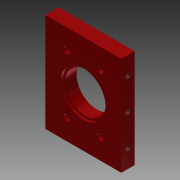
# Autodesk Inventor part: Swerve Wheel + Carriage Outline V1
Saved by Autodesk Inventor 2013 (Build 170138000, 138)
## iProperties
Created: 2013-04-01
Part Number: Swerve Wheel + Carriage Outline V1
Material: Generic
Document SubType Name: Sheet Metal
Designer: mvarma
Density: 1 g/cm^3
Sheet Metal Rule: Default
Author: mvarma
Autodesk Inventor part; units mm, degrees
ref_plane "YZ Plane" through (0, 0, 0) normal (1, 0, 0) x (0, 1, 0)
ref_plane "XZ Plane" through (0, 0, 0) normal (0, 1, 0) x (-1, 0, 0)
sketch "Sketch1" plane through (0, 0, 0) normal (0, 0, 1) x (1, 0, 0)
  circle A0 centre (0, 0) radius 38.1 construction
  circle A1 centre (0, 0) radius 41.275 construction
  line L0 (-7.3323, 0) -> (-3.6662, 6.35) construction
  line L1 (-3.6662, 6.35) -> (3.6662, 6.35) construction
  line L2 (3.6662, 6.35) -> (7.3323, 0) construction
  line L3 (7.3323, 0) -> (3.6662, -6.35) construction
  line L4 (3.6662, -6.35) -> (-3.6662, -6.35) construction
  line L5 (-3.6662, -6.35) -> (-7.3323, 0) construction
  circle A2 centre (0, 0) radius 14.2875 construction
  circle A3 centre (0, 0) radius 15.875 construction
  circle A4 centre (0, 0) radius 8.7313 construction
  circle A5 centre (0, 0) radius 22.225 construction
  line L6 (34.925, 38.1) -> (34.925, 95.25) construction
  line L7 (34.925, 95.25) -> (-34.925, 95.25) construction
  line L8 (-34.925, 95.25) -> (-34.925, 38.1) construction
  line L9 (34.925, 38.1) -> (-34.925, 38.1) construction
  line L10 (34.925, 38.1) -> (21.2491, -6.5137) construction
  line L11 (-34.925, 38.1) -> (-21.2491, -6.5137) construction
  circle A6 centre (-30.353, 38.1) radius 3.9624 construction
  line L12 (53.34, 95.25) -> (-53.34, 95.25) construction
  line L13 (-53.34, 95.25) -> (-53.34, 104.775) construction
  line L14 (-53.34, 104.775) -> (53.34, 104.775) construction
  line L15 (53.34, 104.775) -> (53.34, 95.25) construction
  circle A7 centre (-222.5199, 24.1494) radius 53.34 construction
  line L16 (-190.7699, 59.0744) -> (-254.2699, 59.0744)
  line L17 (-254.2699, 59.0744) -> (-254.2699, -10.7756)
  line L18 (-254.2699, -10.7756) -> (-190.7699, -10.7756)
  line L19 (-190.7699, -10.7756) -> (-190.7699, 59.0744)
  line L20 (-195.5324, 59.0744) -> (-195.5324, -10.7756)
  line L21 (-249.5074, 59.0744) -> (-249.5074, -10.7756)
  line L22 (-209.8199, 68.5994) -> (-235.2199, 68.5994) construction
  line L23 (-235.2199, 68.5994) -> (-235.2199, -20.3006) construction
  line L24 (-235.2199, -20.3006) -> (-209.8199, -20.3006) construction
  line L25 (-209.8199, -20.3006) -> (-209.8199, 68.5994) construction
  line L26 (34.925, 88.9) -> (-34.925, 88.9) construction
  circle A8 centre (30.353, 38.1) radius 3.9624 construction
  circle A9 centre (30.353, 76.2) radius 3.9624 construction
  circle A10 centre (-30.353, 76.2) radius 3.9624 construction
  circle A11 centre (0, 47.625) radius 3.9624 construction
  line L27 (34.925, 92.075) -> (-34.925, 92.075) construction
  circle A12 centre (0, 71.755) radius 14.2875 construction
  circle A13 centre (0, 71.755) radius 15.875 construction
  line L28 (7.3323, 71.755) -> (3.6662, 65.405) construction
  line L29 (3.6662, 65.405) -> (-3.6662, 65.405) construction
  line L30 (-3.6662, 65.405) -> (-7.3323, 71.755) construction
  line L31 (-7.3323, 71.755) -> (-3.6662, 78.105) construction
  line L32 (-3.6662, 78.105) -> (3.6662, 78.105) construction
  line L33 (3.6662, 78.105) -> (7.3323, 71.755) construction
  point P0 (22.225, 92.075)
  point P1 (0, 92.075)
  point P2 (-22.225, 92.075)
  point P3 (0, 47.625)
  dimension "d0" = 76.2
  dimension "d2" = 82.55
  dimension "d3" = 12.7
  dimension "d4" = 28.575
  dimension "d5" = 31.75
  dimension "d6" = 17.4625
  dimension "d7" = 44.45
  dimension "d8" = 69.85
  dimension "d9" = 34.925
  dimension "d10" = 38.1
  dimension "d11" = 57.15
  dimension "d13" = 7.9248
  dimension "d14" = 9.525
  dimension "d15" = 106.68
  dimension "d16" = 53.34
  dimension "d17" = 106.68
  dimension "d18" = 69.85
  dimension "d19" = 34.925
  dimension "d20" = 63.5
  dimension "d21" = 31.75
  dimension "d22" = 4.7625
  dimension "d23" = 4.7625
  dimension "d24" = 25.4
  dimension "d25" = 14.2875
  dimension "d26" = 88.9
  dimension "d27" = 14.2875
  dimension "d28" = 44.45
  dimension "d29" = 4.572
  dimension "d30" = 6.35
  dimension "d31" = 0
  dimension "d32" = 7.9248
  dimension "d33" = 4.572
  dimension "d34" = 7.9248
  dimension "d35" = 7.9248
  dimension "d36" = 4.572
  dimension "d37" = 4.572
  dimension "d38" = 38.1
  dimension "d39" = 38.1
  dimension "d40" = 7.9248
  dimension "d41" = 9.525
  dimension "d42" = 34.925
  dimension "d44" = 3.175
  dimension "d45" = 34.925
  dimension "d46" = 12.7
  dimension "d47" = 12.7
  dimension "d48" = 28.575
  dimension "d50" = 0
  dimension "d52" = 31.75
  dimension "d53" = 12.7
  dimension "d54" = 17.145
  measures "d0" diameter of A0
  measures "d2" diameter of A1
  measures "d3" distance between parallel lines of L4 L1
  measures "d4" diameter of A2
  measures "d5" diameter of A3
  measures "d6" diameter of A4
  measures "d7" diameter of A5
  measures "d8" distance between parallel lines of L8 L6
  measures "d9" distance from line of point (0, 0) L8
  measures "d10" distance from line of L9 point (0, 0)
  measures "d11" distance of L7.end L8.end
  measures "d13" diameter of A6
  measures "d14" distance of L14.end L12.start
  measures "d15" distance of L13.end L14.end
  measures "d16" horizontal distance of L12.start point (0, 0)
  measures "d17" diameter of A7
  measures "d18" distance of L18.end L16.start
  measures "d19" distance from line of A7.centre L18
  measures "d20" distance of L17.end L18.end
  measures "d21" distance from line of L19 A7.centre
  measures "d22" distance between parallel lines of L17 L21
  measures "d23" distance between parallel lines of L19 L20
  measures "d24" distance between parallel lines of L23 L25
  measures "d25" distance between parallel lines of L20 L25
  measures "d26" distance of L22.end L23.end
  measures "d27" distance between parallel lines of L21 L23
  measures "d28" distance from line of A7.centre L24
  measures "d29" distance from line of L8 A6.centre
  measures "d30" distance between parallel lines of L7 L26
  measures "d31" distance between parallel lines of L7 L12
  measures "d32" diameter of A8
  measures "d33" distance from line of L6 A8.centre
  measures "d34" diameter of A9
  measures "d35" diameter of A10
  measures "d36" distance from line of L8 A10.centre
  measures "d37" distance from line of L6 A9.centre
  measures "d38" distance from line of L9 A10.centre
  measures "d39" distance from line of L9 A9.centre
  measures "d40" diameter of A11
  measures "d41" distance from line of L9 A11.centre
  measures "d42" distance from line of L8 A11.centre
  measures "d44" distance between parallel lines of L26 L27
  measures "d45" distance from line of L8 point (0, 92.075)
  measures "d46" distance from line of L8 point (-22.225, 92.075)
  measures "d47" distance from line of L6 point (22.225, 92.075)
  measures "d48" diameter of A12
  measures "d50" horizontal distance of A11.centre A12.centre
  measures "d52" diameter of A13
  measures "d53" distance between parallel lines of L29 L32
  measures "d54" distance from line of L26 A13.centre
extrude "Plate1" add sketch "Sketch1" along normal blind 9.525 contours L20 L18 L21 L16
sketch "Sketch3" plane through (0, 0, 0) normal (0, 0, -1) x (-1, 0, 0)
  line L0 (249.5074, -10.7756) -> (195.5324, -10.7756) projected
  line L1 (249.5074, 59.0744) -> (249.5074, -10.7756) projected
  circle A0 centre (222.5199, 24.1494) radius 23.8125 construction
  line L2 (210.6137, 44.7716) -> (222.5199, 24.1494) construction
  line L3 (222.5199, 24.1494) -> (198.7074, 24.1494) construction
  point P0 (195.5324, 59.0744)
  point P1 (0, 0)
  point P2 (198.7074, 24.1494)
  point P3 (210.6137, 3.5271)
  point P4 (234.4262, 3.5271)
  point P5 (246.3324, 24.1494)
  point P6 (234.4262, 44.7716)
  dimension "d69" = 47.625
  dimension "d71" = 26.9875
  dimension "d72" = 53.975
  dimension "d73" = 34.925
  dimension "d74" = 69.85
  dimension "d75" = 60
  dimension "d78" = 360
  constraints: 4 end point, 2 point on circle, 1 centre point, 1 coincident, 1 perpendicular, 7 other
  measures "d69" diameter of A0
  measures "d71" distance from line of L1 L2.end
  measures "d72" distance of point (195.532, 59.074) L1.start
  measures "d73" distance from line of L0 L2.end
  measures "d74" distance of L1.start L0.start
  measures "d75" angle of L3 L2
hole "Hole2" at (-210.6137, 44.7716, 0) at (-210.6137, 3.5271, 0) at (-234.4262, 3.5271, 0) at (-234.4262, 44.7716, 0) direction (0, 0, 1) diameter 4.318 end through all counterbore diameter 7.9502 counterbore depth 3.175 clearance for "Socket Head Cap Screw" size "#8" standard "Ansi Unified Screw Threads"
sketch "Sketch4" plane through (0, 0, 9.525) normal (0, 0, 1) x (1, 0, 0)
  line L0 (-249.5074, -10.7756) -> (-249.5074, 59.0744) projected
  line L1 (-195.5324, -10.7756) -> (-249.5074, -10.7756) projected
  point P0 (0, 0)
  point P1 (-222.5199, 24.1494)
  dimension "d97" = 53.975
  dimension "d98" = 69.85
  dimension "d99" = 34.925
  dimension "d100" = 26.9875
  measures "d97" distance of L1.start L0.start
  measures "d98" distance of L0.start L0.end
  measures "d99" distance from line of L1 point (-222.52, 24.149)
  measures "d100" distance from line of L0 point (-222.52, 24.149)
hole "Hole4" at (-222.5199, 24.1494, 9.525) direction (0, 0, -1) diameter 28.575 end through all counterbore diameter 31.75 counterbore depth 1.5875
ref_plane "Work Plane1" through (-222.5199, -10.7756, 0) normal (1, 0, 0) x (0, 0, -1)
sketch "Sketch2" plane through (-195.5324, -10.7756, 0) normal (1, 0, 0) x (0, 0, -1)
  line L0 (0, 0) -> (-9.525, 0) projected
  line L1 (0, 69.85) -> (-9.525, 69.85) projected
  line L2 (-4.7625, 69.85) -> (-4.7625, 0) construction
  point P0 (0, 10.7756)
  point P1 (-4.7625, 57.15)
  point P2 (-4.7625, 34.925)
  point P3 (-4.7625, 12.7)
  dimension "d87" = 12.7
  dimension "d88" = 12.7
  dimension "d89" = 34.925
  constraints: 3 midpoint, 2 end point, 2 point on line
  measures "d87" distance from line of L1 point (-4.763, 57.15)
  measures "d88" distance from line of L0 point (-4.763, 12.7)
  measures "d89" distance from line of L0 point (-4.763, 34.925)
hole "Hole1" at (-195.5324, 46.3744, 4.7625) at (-195.5324, 24.1494, 4.7625) at (-195.5324, 1.9244, 4.7625) direction (-1, 0, 0) diameter 3.9624 depth 7.9375 tip angle 118 thread size "10-32 UNF" class "2B" standard "ANSI Unified Screw Threads"
mirror "Mirror1" about plane through (-222.5199, -10.7756, 0) normal (1, 0, 0) of "Hole1"
equation "\"d99\" = 0.5 * d98"
equation "\"d100\" = 0.5 * d97"
equation "\"d9\" = 0.5 * d8"
equation "\"d16\" = 0.5 * d15"
equation "\"d19\" = 0.5 * d18"
equation "\"d21\" = 0.5 * d20"
equation "\"d22\" = d23"
equation "\"d25\" = d27"
equation "\"d28\" = 0.5 * d26"
equation "\"d32\" = d13"
equation "\"d33\" = d29"
equation "\"d34\" = d32"
equation "\"d35\" = d13"
equation "\"d36\" = d29"
equation "\"d37\" = d29"
equation "\"d39\" = d38"
equation "\"d40\" = d13"
equation "\"d44\" = 0.5 * d30"
equation "\"d71\" = 0.5 * d72"
equation "\"d73\" = 0.5 * d74"
equation "\"d106\" = Thickness"
equation "\"d45\" = d42"
equation "\"d47\" = d46"
equation "\"BendRadius\" = Thickness"
equation "\"BendReliefWidth\" = Thickness"
equation "\"BendReliefDepth\" = 0.5 * Thickness"
equation "\"CornerReliefSize\" = 4 * Thickness"
equation "\"MinimumRemnant\" = 2 * Thickness"
equation "\"TransitionRadius\" = BendRadius"
equation "\"JacobiRadiusSize\" = Thickness"
equation "\"GapSize\" = Thickness"
equation "\"d55\" = BendRadius"
equation "\"Thickness\" = 9.525"
body "Solid1"
